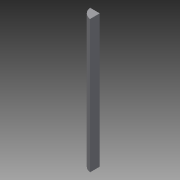
# Autodesk Inventor part: styroFoamMandrel
Saved by Autodesk Inventor 2014 (Build 180170000, 170)
## iProperties
Created: 2014-02-10
Part Number: styroFoamMandrel
Material: Generic
Document SubType Name: Modeling
Designer: clang
Density: 1 g/cm^3
Appearance: Default
Author: clang
Autodesk Inventor part; units mm, degrees
ref_plane "YZ Plane" through (0, 0, 0) normal (1, 0, 0) x (0, 1, 0)
ref_plane "XZ Plane" through (0, 0, 0) normal (0, 1, 0) x (-1, 0, 0)
ref_plane "XY Plane" through (0, 0, 0) normal (0, 0, 1) x (1, 0, 0)
sketch "Sketch1" plane through (0, 0, 0) normal (0, 1, 0) x (-1, 0, 0)
  arc A0 (105.8221, 15.9999) -> (16.0001, 105.822) centre (0, 0) ccw
  line L0 (16.0001, 16.0002) -> (105.8221, 15.9999)
  line L1 (16.0001, 105.822) -> (16.0001, 16.0002)
  arc A1 (105.8221, 15.9999) -> (16.0001, 105.822) centre (0, 0) ccw
  line L2 (16.0001, 16.0002) -> (105.8221, 15.9999)
  line L3 (16.0001, 105.822) -> (16.0001, 16.0002)
  dimension "d2" = 180
  constraints: 8 end point, 4 point on circle, 2 centre point, 1 coincident, 8 other
extrude "Extrusion1" add sketch "Sketch1" along normal blind 1219.2
body "Solid1"
